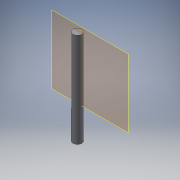
# Autodesk Inventor part: Motor-Shaft
Saved by Autodesk Inventor 2019 (Build 230136000, 136)
## iProperties
Created: 2021-01-03
Part Number: Motor-Shaft
Material: Generic
Document SubType Name: Modeling
Designer: Sam
Density: 1 g/cm^3
Appearance: Default
Author: Sam
Autodesk Inventor part; units mm, degrees
ref_plane "YZ Plane" through (0, 0, 0) normal (1, 0, 0) x (0, 1, 0)
ref_plane "XZ Plane" through (0, 0, 0) normal (0, 1, 0) x (-1, 0, 0)
ref_plane "XY Plane" through (0, 0, 0) normal (0, 0, 1) x (1, 0, 0)
ref_plane "Work Plane1" through (0, -7.6831, 0) normal (0, 0, 1) x (-1, 0, 0)
sketch "Sketch1" plane through (0, -7.6831, 0) normal (0, 0, 1) x (-1, 0, 0)
  line L0 (0, -7.6831) -> (0, 31.0323)
  line L1 (0, -7.6831) -> (1.5, -7.6831)
  line L2 (1.5, -7.6831) -> (1.5, 24.3169)
  line L3 (1.5, 24.3169) -> (0, 24.3169)
  line L4 (0, 24.3169) -> (0, -7.6831)
  dimension "d0" = 32
  dimension "d1" = 3
  constraints: 10 end point, 2 perpendicular, 1 collinear, 1 horizontal, 1 vertical
  measures "d0" distance of L1.end L2.end
  measures "d1" diameter of L2 L0
revolve "Revolution1" add sketch "Sketch1" angle 360 about axis through (0, 0, 0) along (0, -1, 0)
sketch "Sketch2" plane through (0, -32, 0) normal (0, -1, 0) x (1, 0, 0)
  circle A0 centre (0, 0) radius 1.5 projected
  line L0 (-1, -1.118) -> (-1, 1.118)
  point P0 (0, 0)
  dimension "d3" = 1
  constraints: 2 end point, 2 point on circle, 1 vertical
  measures "d3" distance from line of point (0, 0) L0
extrude "Extrusion1" cut sketch "Sketch2" against normal blind 9.3 contours L0 A0 picked at (-1.1631, -0.0599)
body "Solid1"
